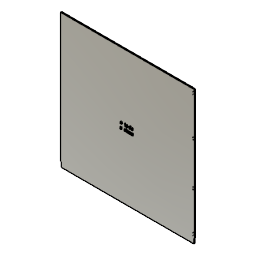
3X8X_Door_v3_2025_11_20 (Autodesk Fusion 360 design; units mm, degrees)
part number: Configuration 1
Autodesk Fusion 360 part; units mm, degrees
note: some values were not read from the file. Chosen so that the rebuilt part matches the saved one: which bodies a step acts on.
sketch "MasterSketch" plane through (0, 0, 0) normal (0, 1, 0) x (1, 0, 0)
  line L0 (-1168.4, -2362.2) -> (1168.4, -2362.2)
  line L1 (1168.4, -2362.2) -> (1168.4, -25.4)
  line L2 (1168.4, -25.4) -> (-1168.4, -25.4)
  line L3 (-1168.4, -25.4) -> (-1168.4, -2362.2)
  line L4 (0, -25.4) -> (0, 0) construction
  line L5 (1143.8128, -2362.2) -> (1143.8128, -25.4) construction
  circle A0 centre (1143.8128, -2318.512) radius 6.35
  circle A1 centre (1143.8128, -2280.412) radius 6.35
  circle A2 centre (1143.8128, -153.162) radius 6.35
  circle A3 centre (1143.8128, -191.262) radius 6.35
  circle A4 centre (1143.8128, -1592.2329) radius 6.35
  circle A5 centre (1143.8128, -1630.3329) radius 6.35
  circle A6 centre (1143.8128, -841.3411) radius 6.35
  circle A7 centre (1143.8128, -879.4411) radius 6.35
  line L6 (-1160.78, -2362.2) -> (-1160.78, -25.4)
  line L7 (1160.78, -25.4) -> (1160.78, -2362.2)
  line L8 (1157.1884, -25.4) -> (1157.1884, -109.474)
  line L9 (1157.1884, -109.474) -> (1168.4, -109.474)
  line L10 (-1157.1884, -25.4) -> (-1157.1884, -109.474)
  line L11 (-1157.1884, -109.474) -> (-1168.4, -109.474)
  dimension "d10" = 25.4
  dimension "d11" = 2336.8
  dimension "d12" = 2336.8
  dimension "d24" = 6.35
  dimension "d26" = 43.688
  dimension "d27" = 6.35
  dimension "d30" = 6.35
  dimension "d32" = 6.35
  dimension "d38" = 2312.2128
  dimension "d42" = 24.5872
  dimension "d45" = 7.62
  dimension "d46" = 7.62
  dimension "d55" = 84.074
  dimension "d56" = 11.2116
  dimension "d101" = 81.788
  dimension "d102" = 731.8671
  dimension "d103" = 769.9671
  dimension "d104" = 1482.7589
  dimension "d105" = 1520.8589
  dimension "d106" = 2170.938
  dimension "d107" = 2209.038
  constraint horizontal L0
  constraint vertical L1
  constraint horizontal L2
  constraint vertical L3
  constraint midpoint L2 L4.start
  constraint coincident L4.end origin
  constraint vertical L4
  constraint coincident L0 L5.start
  constraint coincident L2 L5.end
  constraint perpendicular L2 L5
  constraint coincident L5 A0.centre
  constraint coincident L5 A1.centre
  constraint equal A0 A1
  constraint equal A2 A3
  constraint coincident L5 A3.centre
  constraint coincident L5 A2.centre
  constraint equal A4 A5
  constraint equal A6 A7
  constraint coincident L5 A5.centre
  constraint coincident L5 A4.centre
  constraint coincident L5 A7.centre
  constraint coincident L5 A6.centre
  constraint coincident L0 L6.start
  constraint coincident L2 L6.end
  constraint perpendicular L2 L6
  constraint coincident L2 L7.start
  constraint coincident L0 L7.end
  constraint perpendicular L0 L7
  constraint coincident L2 L8.start
  constraint perpendicular L2 L8
  constraint perpendicular L7 L9
  constraint coincident L1 L9.end
  constraint symmetric L4 L8.start L10.start
  constraint symmetric L4 L8.end L10.end
  constraint symmetric L4 L9.end L11.end
  measures "d10" distance of L4.start L4.end
  measures "d11" distance of L0.start L2.end
  measures "d12" distance of L1.end L2.end
  measures "d24" radius of A0
  measures "d26" distance of L0 A0.centre
  measures "d27" radius of A3
  measures "d30" radius of A5
  measures "d32" radius of A7
  measures "d38" distance of L3 L5
  measures "d42" distance of L1.end L5
  measures "d45" distance of L1 L7
  measures "d46" distance of L3 L6
  measures "d55" distance of L8.start L8.end
  measures "d56" distance of L1 L8
  measures "d101" distance of L0 A1.centre
  measures "d102" distance of L0 A5.centre
  measures "d103" distance of L0 A4.centre
  measures "d104" distance of L0 A7.centre
  measures "d105" distance of L0 A6.centre
  measures "d106" distance of L0 A3.centre
  measures "d107" distance of L0 A2.centre
extrude "door_extrude" add sketch "MasterSketch" along normal mid plane 19.05 contours L0 L3 L6 L11 | L0 L2 L6 L7 L8 L9 L10 L11 | L2 L3 L6 L11 | L0 L1 L7 L9 | L2 L6 L10 L11 | L2 L7 L8 L9 | L1 L2 L7 L9 | A0 | A1 | A2 | A3 | A4 | A5 | A6 | A7 makes body 1 in component "door_panel"
extrude "routing_Left" add sketch "MasterSketch" along normal blind 12.7 from surface at 9.525 separate body contours L0 L3 L6 L11 | L2 L3 L6 L11 makes body 2 in component "door_panel"
extrude "Extrude6" add sketch "MasterSketch" against normal blind 12.7 from surface at 9.525 separate body contours L0 L1 L7 L9 | L1 L2 L7 L9 makes body 3 in component "door_panel"
combine "Combine2" operation cut target body 1 tool bodies 2 3 in component "door_panel"
extrude "hinge_holes_extrusion" cut sketch "MasterSketch" along normal blind 14.2875 from surface at -9.525 contours A0 | A1 | A2 | A3 | A4 | A5 | A6 | A7 bodies 1 in component "door_panel"
extrude "door_notch_left" add sketch "MasterSketch" along normal blind 19.05 from surface at -9.525 separate body contours L2 L3 L6 L11 | L2 L6 L10 L11 makes body 4 in component "door_panel"
extrude "doo_notch_right" add sketch "MasterSketch" along normal blind 19.05 from surface at -9.525 separate body contours L2 L7 L8 L9 | L1 L2 L7 L9 makes body 5 in component "door_panel"
combine "notch_cut" operation cut target body 1 tool bodies 4 5 in component "door_panel"
sketch "Labels" plane through (0, 0, 0) normal (0, 1, 0) x (1, 0, 0)
  line L0 (1168.4, -25.4) -> (-1168.4, -2362.2) construction
  line L1 (1168.4, -2362.2) -> (-1168.4, -25.4) construction
  line L2 (-139.7, -1117.6) -> (139.7, -1117.6) construction
  line L3 (139.7, -1117.6) -> (139.7, -1270) construction
  line L4 (139.7, -1270) -> (-139.7, -1270) construction
  line L5 (-139.7, -1270) -> (-139.7, -1117.6) construction
  line L6 (139.7, -1117.6) -> (-139.7, -1270) construction
  line L7 (-139.7, -1117.6) -> (139.7, -1117.6) construction
  line L8 (139.7, -1117.6) -> (139.7, -1270) construction
  line L9 (139.7, -1270) -> (-139.7, -1270) construction
  line L10 (-139.7, -1270) -> (-139.7, -1117.6) construction
  point P0 (-1168.4, -2362.2)
  point P1 (1168.4, -2362.2)
  point P2 (1168.4, -25.4)
  point P3 (-1168.4, -25.4)
  point P4 (0, -1193.8)
  dimension "d74" = 50.8
  dimension "d76" = 279.4
  dimension "d77" = 152.4
  dimension "d78" = 50.8
  text T0 "inside the stall" font "Arial" height 50.8 align centre top in box 279.4 x 152.4 at (-139.7, -1117.6) x (1, 0) y (0, -1) spacing 1
  text T1 "outside surface" font "Arial" height 50.8 align centre top in box 279.4 x 152.4 at (-139.7, -1117.6) x (1, 0) y (0, -1) spacing 1
  constraint coincident P2 L0.start
  constraint coincident P0 L0.end
  constraint coincident P1 L1.start
  constraint coincident P3 L1.end
  constraint coincident L0 P4
  constraint coincident L1 P4
  constraint coincident L2.end
  constraint coincident L4.end
  constraint midpoint P4 L6
  constraint horizontal L4
  constraint horizontal L9
  constraint collinear L5 L10
  constraint collinear L3 L8
  constraint collinear L2 L7
  constraint collinear L4 L9
extrude "Extrude1" add sketch "Labels" against normal mid plane 6.35 from surface at -25.4 separate body text T1 makes body 6 at (49.5025, -28.575, 1147.1814) makes body 7 at (-9.1597, -28.575, 1150.5657) makes body 8 at (-94.3116, -28.575, 1158.8762) makes body 9 at (100.4911, -28.575, 1237.7158) makes body 10 at (26.89, -28.575, 1243.7337) makes body 11 at (6.2835, -28.575, 1238.1603) makes body 12 at (-42.2756, -28.575, 1237.1613) makes body 13 at (-25.1459, -28.575, 1236.9188) makes body 14 at (26.89, -28.575, 1267.609) makes body 15 at (68.2455, -28.575, 1243.3881) makes body 16 at (-109.358, -28.575, 1240.1432) makes body 17 at (-48.2011, -28.575, 1157.8773) makes body 18 at (34.662, -28.575, 1150.3629) makes body 19 at (102.4317, -28.575, 1158.4317) in component "OutLabel"
extrude "Extrude2" add sketch "Labels" against normal blind 6.35 from surface at 25.4 separate body text T0 makes body 20 at (-86.1278, 21.1667, 1243.7337) makes body 21 at (-13.9361, 25.4, 1238.1603) makes body 22 at (4.5914, 21.1667, 1243.7337) makes body 23 at (80.2716, 25.4, 1237.7158) makes body 24 at (-110.4594, 25.4, 1157.6347) makes body 25 at (-36.0729, 25.4, 1158.4317) makes body 26 at (43.396, 25.4, 1157.6347) makes body 27 at (97.1645, 21.1667, 1173.7826) makes body 28 at (85.4967, 25.4, 1150.3629) makes body 29 at (19.6245, 25.4, 1158.8762) makes body 30 at (-93.9247, 25.4, 1164.2022) makes body 31 at (112.9312, 21.1667, 1173.7826) makes body 32 at (48.026, 25.4, 1243.3881) makes body 33 at (4.5914, 21.1667, 1265.218) makes body 34 at (-68.3166, 25.4, 1238.1663) makes body 35 at (-86.1278, 21.1667, 1265.218)
copy_body "CutPasteBodies1" bodies 20 25 26 21 22 28 29 32 24 31 27 33 35 30 34 23 removing the originals makes body 36 makes body 37 makes body 38 makes body 39 makes body 40 makes body 41 makes body 42 makes body 43 makes body 44 makes body 45 makes body 46 makes body 47 makes body 48 makes body 49 makes body 50 makes body 51 in component "InLabel"
fillet "Fillet1" radius 6.35 2 edges at (-1157.1884, 0, 109.474) (1157.1884, 0, 109.474) on bodies 1 in component "door_panel"
component "door_panel" placed x (1, 0, 0) y (0, 1, 0) z (0, 0, 1) at (0, 0, 0)
component "OutLabel" placed x (1, 0, 0) y (0, 1, 0) z (0, 0, 1) at (0, 0, 0)
component "InLabel" placed x (1, 0, 0) y (0, 1, 0) z (0, 0, 1) at (0, 0, 0)
equation "component_height = 92 in" comment "000) Input - Model     Height of the component"
equation "component_width = 92 in" comment "001) Input - Model     Width of the component"
equation "component_floor_clearance = 1 in" comment "002) Input - Model     Floor clearance of the component"
equation "door_hinging_right = 1" comment "003) Input - Model     Whether the door's hinges are on the right side of the door"
equation "d10 = component_floor_clearance"
equation "d11 = component_height"
equation "d12 = component_width"
equation "hinge_hole_radius = 0.25 in" comment "016) Fixed - Model     The radius of the hinge holes"
equation "component_thickness = 0.75 in" comment "017) Fixed - Model     The thickness of the component"
equation "door_top_margin = 1.72 in" comment "011) Fixed - Helper     Distance between top-most hole and top of door"
equation "door_bottom_margin = 1.72 in + if(( component_floor_clearance == 1 in ) and not(door_wall_post_hinging); notching_y_dist; 0 in)" comment "012) Derived - Helper     Distance between bottom-most hole and bottom of door"
equation "door_swinging_out = 1" comment "004) Input - Model     Whether the door is an outswing door"
equation "door_wall_post_hinging = 0" comment "005) Input - Model     Whether the door hinges on a wall post"
equation "door_wall_keep_latching = 0" comment "006) Input - Model     Whether the door latches on a wall keep"
equation "notching_x_dist = 0.4414 in" comment "018) Fixed - Model     The horizontal width of the notching"
equation "notching_y_dist = 3.31 in" comment "009) Fixed - Model     Height of notching cutout from bottom of door"
equation "hinge_hole_space = 1.5 in" comment "013) Fixed - Helper     Distance between the top and bottom hole on a single hinge"
equation "d24 = hinge_hole_radius"
equation "d26 = top_hinge_hole_1_y_value"
equation "d27 = hinge_hole_radius"
equation "d30 = hinge_hole_radius"
equation "d32 = hinge_hole_radius"
equation "hinge_hole_x_dist = 0.968 in" comment "008) Fixed - Model     Horizontal distance between hinge holes and edge of stile"
equation "d38 = hole_placement"
equation "d39 = component_thickness"
equation "hole_placement = if(left_exterior_drilling or right_interior_drilling; hinge_hole_x_dist; component_width - hinge_hole_x_dist)" comment "105) Derived - Model     An offset that shifts the hinge holes to the appropriate side of the component"
equation "rabbeting_width = 0.3 in" comment "019) Fixed - Model     The horizontal width of the rabbeting"
equation "rabbeting_depth = 0.5 in" comment "020) Fixed - Model     The depth of the rabbeting"
equation "d45 = rabbeting_width"
equation "d46 = rabbeting_width"
equation "d48 = left_rabbeting_model"
equation "hinge_hole_depth = 0.5625 in" comment "021) Fixed - Model     The depth of the hinge holes"
equation "d51 = hinge_hole_depth"
equation "d55 = notching_y_dist"
equation "d56 = notching_x_dist"
equation "d59 = if(left_notching; component_thickness; -component_thickness)"
equation "left_notching = if(not(component_floor_clearance == 1 in); 0; if(( left_interior_drilling or left_exterior_drilling ) and door_wall_post_hinging; 0; if(( right_interior_drilling or right_exterior_drilling ) and door_wall_keep_latching; 0; 1)))" comment "301) Derived - Model     Whether the bottom left corner of the door is notched to accommodate the shoe on a stile"
equation "right_notching = if(not(component_floor_clearance == 1 in); 0; if(( right_interior_drilling or right_exterior_drilling ) and door_wall_post_hinging; 0; if(( left_interior_drilling or left_exterior_drilling ) and door_wall_keep_latching; 0; 1)))" comment "302) Derived - Model     Whether the bottom right corner of the door is notched to accommodate the shoe on a stile"
equation "d71 = if(right_notching; component_thickness; -component_thickness)"
equation "d75 = 'inside the stall'"
equation "d79 = 'outside surface'"
equation "d82 = label_out_positioning_offset"
equation "label_out_positioning_offset = ( if(not(door_swinging_out); -1; 1) ) * 1 in" comment "023) Derived - Model     Calculates the placement of label tag"
equation "label_in_positioning_offset = ( if(not(door_swinging_out); 1; -1) ) * 1 in" comment "022) Derived - Model     Calculates the placement of label tag"
equation "d87 = label_in_positioning_offset"
equation "top_hinge_hole_1_y_value = door_top_margin" comment "401) Derived - Model     Distance between top of the door and the center of the door hinge hole"
equation "top_hinge_hole_2_y_value = top_hinge_hole_1_y_value + hinge_hole_space" comment "402) Derived - Model     Distance between top of the door and the center of the door hinge hole"
equation "inter_hinge_gap = ( component_height - ( door_top_margin ) - ( door_bottom_margin + hinge_hole_space ) ) / 3" comment "010) Derived - Helper     Distance between top holes of adjacent hinges"
equation "mid_top_hinge_offset = ( -1 * 0.823 * if(component_floor_clearance == 1 in and not(door_wall_post_hinging); 1; 0) ) * 1 in" comment "014) Derived - Helper     An offset applying to the mid-top hinge when the floor clearance is 1\"\" the door hinges on a stile"
equation "mid_top_hinge_hole_1_y_value = top_hinge_hole_1_y_value + inter_hinge_gap + mid_top_hinge_offset" comment "403) Derived - Model     Distance between top of the door and the center of the door hinge hole"
equation "mid_top_hinge_hole_2_y_value = mid_top_hinge_hole_1_y_value + hinge_hole_space" comment "404) Derived - Model     Distance between top of the door and the center of the door hinge hole"
equation "mid_bottom_hinge_offset = ( 2 * 0.823 * if(component_floor_clearance == 1 in and not(door_wall_post_hinging); 1; 0) ) * 1 in" comment "015) Derived - Helper     An offset applying to the mid-bottom hinge when the floor clearance is 1\"\" the door hinges on a stile"
equation "mid_bottom_hinge_hole_1_y_value = mid_top_hinge_hole_1_y_value + inter_hinge_gap + mid_bottom_hinge_offset" comment "405) Derived - Model     Distance between top of the door and the center of the door hinge hole"
equation "mid_bottom_hinge_hole_2_y_value = mid_bottom_hinge_hole_1_y_value + hinge_hole_space" comment "406) Derived - Model     Distance between top of the door and the center of the door hinge hole"
equation "bottom_hinge_hole_1_y_value = mid_bottom_hinge_hole_1_y_value + inter_hinge_gap + mid_top_hinge_offset" comment "407) Derived - Model     Distance between top of the door and the center of the door hinge hole"
equation "bottom_hinge_hole_2_y_value = bottom_hinge_hole_1_y_value + hinge_hole_space" comment "408) Derived - Model     Distance between top of the door and the center of the door hinge hole"
equation "d101 = top_hinge_hole_2_y_value"
equation "d102 = mid_top_hinge_hole_1_y_value"
equation "d103 = mid_top_hinge_hole_2_y_value"
equation "d104 = mid_bottom_hinge_hole_1_y_value"
equation "d105 = mid_bottom_hinge_hole_2_y_value"
equation "d106 = bottom_hinge_hole_1_y_value"
equation "d107 = bottom_hinge_hole_2_y_value"
equation "door_perp_stile_keeper = 1" comment "007) Input - Model     Whether the door latches on a perpendiculat stile"
equation "left_rabbeting_model = if(right_exterior_rabbeting or left_interior_rabbeting; -rabbeting_depth; rabbeting_depth)" comment "203) Derived - Model     Controls rabbeting in model's left side as seen from the FRONT"
equation "right_rabbeting_model = if(left_exterior_rabbeting or right_interior_rabbeting; -rabbeting_depth; rabbeting_depth)" comment "206) Derived - Model     Controls rabbeting in model's right side as seen from the FRONT"
equation "d114 = right_rabbeting_model"
equation "left_interior_drilling = if(not(door_hinging_right) and not(door_swinging_out); 1; 0)" comment "101) Derived - Model     Whether drilling is present the interior left edge of the door"
equation "left_exterior_drilling = if(not(door_hinging_right) and door_swinging_out; 1; 0)" comment "102) Derived - Model     Whether drilling is present the exterior left edge of the door"
equation "right_interior_drilling = if(door_hinging_right and not(door_swinging_out); 1; 0)" comment "103) Derived - Model     Whether drilling is present the interior right edge of the door"
equation "right_exterior_drilling = if(door_hinging_right and door_swinging_out; 1; 0)" comment "104) Derived - Model     Whether drilling is present the exterior right edge of the door"
equation "left_interior_rabbeting = if(door_swinging_out and ( not(door_hinging_right) or ( door_hinging_right and not(door_wall_keep_latching or door_perp_stile_keeper) ) ); 1; 0)" comment "201) Derived - Model     Whether routing is present the interior left edge of the door"
equation "left_exterior_rabbeting = if(not(door_swinging_out) and ( not(door_hinging_right) or ( door_hinging_right and not(door_wall_keep_latching or door_perp_stile_keeper) ) ); 1; 0)" comment "202) Derived - Model     Whether routing is present the exterior left edge of the door"
equation "right_interior_rabbeting = if(door_swinging_out and ( door_hinging_right or ( not(door_hinging_right) and not(door_wall_keep_latching or door_perp_stile_keeper) ) ); 1; 0)" comment "204) Derived - Model     Whether rabbeting is present the interior right edge of the stile"
equation "right_exterior_rabbeting = if(not(door_swinging_out) and ( door_hinging_right or ( not(door_hinging_right) and not(door_wall_keep_latching or door_perp_stile_keeper) ) ); 1; 0)" comment "205) Derived - Model     Whether rabbeting is present the exterior right edge of the stile"
named bodies: "door_panel", "left_notch", "right_notch", "LeftRout", "RightRout"
